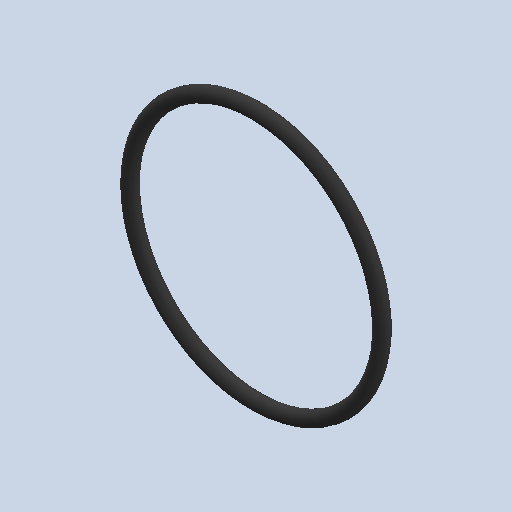
# Autodesk Inventor part: pld-vessel-gasket
Saved by Autodesk Inventor 2026 (Build 300175050, 175E)
## iProperties
Created: 2025-11-13
Part Number: pld-vessel-gasket
Material: Rubber
Document SubType Name: Modeling
Designer: kuzmin
Density: 0.93 g/cm^3
Appearance: Rubber - Black
Author: kuzmin
Autodesk Inventor part; units mm, degrees
ref_plane "YZ Plane" through (0, 0, 0) normal (1, 0, 0) x (0, 1, 0)
ref_plane "XZ Plane" through (0, 0, 0) normal (0, 1, 0) x (-1, 0, 0)
ref_plane "XY Plane" through (0, 0, 0) normal (0, 0, 1) x (1, 0, 0)
sketch "Sketch1" plane through (0, 0, 0) normal (0, 1, 0) x (-1, 0, 0)
  circle A0 centre (-31.5, 0) radius 1.75
  line L0 (0, 0) -> (0, 14.6099)
  dimension "d0" = 3.5
  dimension "d1" = 63
  constraints: 2 end point, 1 centre point, 1 vertical
  measures "d0" diameter of A0
  measures "d1" diameter of A0.centre L0
revolve "Revolution1" add sketch "Sketch1" angle 360 about axis through (0, 0, 0) along (0, 0, 1)
equation "\"d0\" = oring"
equation "\"d1\" = diameter"
equation "\"diameter\" = 63"
equation "\"oring\" = 3.5"
body "Solid1"
